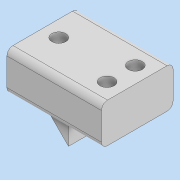
# Autodesk Inventor part: 22_Blocco_Escursione_Braccio
Saved by Autodesk Inventor 2020 (Build 240168000, 168)
## iProperties
Created: 2019-11-16
Part Number: 22_Blocco_Escursione_Braccio
Material: Generico
Document SubType Name: Modeling
Designer: socci
Density: 1 g/cm^3
Appearance: Default
Author: socci
Autodesk Inventor part; units mm, degrees
ref_plane "YZ Plane" through (0, 0, 0) normal (1, 0, 0) x (0, 1, 0)
ref_plane "XZ Plane" through (0, 0, 0) normal (0, 1, 0) x (-1, 0, 0)
ref_plane "XY Plane" through (0, 0, 0) normal (0, 0, 1) x (1, 0, 0)
sketch "Schizzo1" plane through (0, 0, 0) normal (0, 1, 0) x (-1, 0, 0)
  line L0 (14.2727, -129.2727) -> (-32.7273, -129.2727)
  line L1 (-32.7273, -129.2727) -> (-32.7273, -164.8727)
  line L2 (-32.7273, -164.8727) -> (14.2727, -164.8727)
  line L3 (14.2727, -164.8727) -> (14.2727, -129.2727)
  line L4 (14.2727, -129.2727) -> (-32.7273, -164.8727) construction
  line L5 (-32.7273, -129.2727) -> (14.2727, -164.8727) construction
  point P0 (0, 0)
  point P1 (-9.2273, -147.0727)
  dimension "d0" = 35.6
  dimension "d1" = 47
  constraints: 12 end point, 2 midpoint, 2 parallel, 1 horizontal, 1 perpendicular
  measures "d0" distance of L0.end L1.end
  measures "d1" distance of L0.start L0.end
extrude "Estrusione1" add sketch "Schizzo1" along normal blind 19.6
sketch "Schizzo2" plane through (0, 0, 0) normal (0, -1, 0) x (1, 0, 0)
  line L0 (-14.2727, -129.2727) -> (32.7273, -129.2727) projected
  line L1 (32.7273, -129.2727) -> (32.7273, -164.8727) projected
  line L2 (32.7273, -129.2727) -> (32.7273, -164.8727)
  line L3 (32.7273, -147.0727) -> (24.7273, -147.0727)
  line L4 (32.7273, -147.0727) -> (24.7273, -147.0727) construction
  line L5 (24.7273, -147.0727) -> (52.7273, -147.0727) construction
  line L6 (24.7273, -147.0727) -> (24.7273, -154.0727)
  line L7 (24.7273, -147.0727) -> (31.7273, -147.0727) construction
  line L8 (24.7273, -147.0727) -> (24.7273, -140.0727)
  line L9 (24.7273, -147.0727) -> (31.7273, -147.0727) construction
  point P0 (0, 0)
  point P1 (0.7273, -147.0727)
  dimension "d4" = 8
  dimension "d5" = 180
  dimension "d19" = 7
  dimension "d20" = 90
  dimension "d21" = 7
  dimension "d22" = 90
  constraints: 16 end point, 5 horizontal, 3 coincident, 3 equal length, 2 vertical, 1 collinear, 1 midpoint
  measures "d4" distance of L3.start L3.end
  measures "d5" angle of L3 L4
  measures "d19" distance of L6.start L6.end
  measures "d20" angle of L6 L7
  measures "d21" distance of L6.start L8.end
  measures "d22" angle of L9 L8
hole "Foro1" at (24.7273, 0, -140.0727) at (24.7273, 0, -154.0727) direction (0, 1, 0) diameter 7 end through all clearance for "Vite a testa piana" size "M6" standard "ANSI - Profilo M Metrico"
fillet "Raccordo1" radius 3 1 edges at (9.2273, 19.6, -129.2727)
fillet "Raccordo2" radius 3 1 edges at (9.2273, 19.6, -164.8727)
fillet "Raccordo3" radius 3 1 edges at (9.2273, 0, -164.8727)
fillet "Raccordo4" radius 3 1 edges at (9.2273, 0, -129.2727)
sketch "Schizzo3" plane through (0, 19.6, 0) normal (0, 1, 0) x (1, 0, 0)
  line L0 (32.7273, 147.0727) -> (-6.2727, 147.0727)
  line L1 (32.7273, 147.0727) -> (71.7273, 147.0727) construction
  line L2 (32.7273, 132.2727) -> (32.7273, 161.8727) projected
  point P0 (0, 0)
  dimension "d23" = 39
  dimension "d24" = 180
  constraints: 4 end point, 2 horizontal, 1 coincident, 1 collinear, 1 midpoint
  measures "d23" distance of L0.start L0.end
  measures "d24" angle of L0 L1
hole "Foro2" at (-6.2727, 19.6, -147.0727) direction (0, -1, 0) diameter 7 end through all clearance for "Vite a testa piana" size "M6" standard "ANSI - Profilo M Metrico"
sketch "Schizzo4" plane through (0, 0, 0) normal (0, -1, 0) x (1, 0, 0)
  line L0 (32.7273, -132.2727) -> (32.7273, -161.8727) projected
  line L1 (8, -215) -> (39.6, -215) construction
  line L2 (13.3273, -161.8727) -> (13.3273, -132.2727)
  line L3 (13.3273, -161.8727) -> (13.3273, -132.2727)
  line L4 (13.3273, -132.2727) -> (3.3273, -132.2727)
  line L5 (3.3273, -132.2727) -> (3.3273, -161.8727)
  line L6 (3.3273, -161.8727) -> (13.3273, -161.8727)
  line L7 (32.7273, -132.2727) -> (-14.2727, -132.2727) projected
  line L8 (78, -150) -> (86, -150) construction
  line L9 (32.7273, -147.0727) -> (24.7273, -147.0727)
  line L10 (32.7273, -147.0727) -> (40.7273, -147.0727) construction
  line L11 (24.7273, -147.0727) -> (13.3273, -147.0727)
  line L12 (24.7273, -147.0727) -> (36.1273, -147.0727) construction
  point P0 (0, 0)
  dimension "d35" = 29.6
  dimension "d36" = 10
  dimension "d44" = 8
  dimension "d45" = 180
  dimension "d46" = 11.4
  dimension "d47" = 180
  constraints: 22 end point, 6 horizontal, 3 parallel, 2 collinear, 2 midpoint, 2 perpendicular
  measures "d35" distance of L2.start L2.end
  measures "d36" distance of L4.end L2.end
  measures "d44" distance of L9.start L9.end
  measures "d45" angle of L9 L10
  measures "d46" distance of L11.end L9.end
  measures "d47" angle of L11 L12
extrude "Estrusione2" add sketch "Schizzo4" along normal blind 10 contours L2 L6 L5 L4
sketch "Schizzo5" plane through (3.3273, 0, -132.2727) normal (0, 0, 1) x (1, 0, 0)
  line L0 (10, 0) -> (10, -10) projected
  line L1 (10, 0) -> (0, 0) projected
  line L2 (10, -10) -> (0, 0)
  line L3 (0, -10) -> (10, -10) projected
  line L4 (0, 0) -> (0, -10) projected
  line L5 (10, -10) -> (0, -10)
  line L6 (0, -10) -> (0, 0)
  point P0 (-3.3273, 0)
  constraints: 6 end point, 2 perpendicular
extrude "Estrusione3" cut sketch "Schizzo5" against normal through all contours L3 L4 L2
fillet "Raccordo5" radius 5 1 edges at (3.3273, 0, -147.0727)
